Autodesk Inventor part; units mm, degrees
(part 5 of 5)
  line L3248 (77.264, 12.2136) -> (77.264, 9.6132) projected
  line L3249 (77.264, 9.6132) -> (78.0881, 9.6132) projected
  line L3250 (53.0271, 16.9127) -> (66.8267, 16.9127) projected
  line L3251 (66.8267, 16.9127) -> (66.8267, 3.113) projected
  line L3252 (53.0271, 3.113) -> (53.0271, 16.9127) projected
  line L3253 (66.8267, 3.113) -> (53.0271, 3.113) projected
  line L3254 (78.0881, 9.6132) -> (78.0881, 3.3431) projected
  line L3255 (78.7329, 22.163) -> (64.9333, 22.163) projected
  line L3256 (78.7329, 35.9625) -> (78.7329, 22.163) projected
  line L3257 (64.9333, 35.9625) -> (78.7329, 35.9625) projected
  line L3258 (69.2079, 41.2129) -> (55.4083, 41.2129) projected
  line L3259 (69.2079, 55.0125) -> (69.2079, 41.2129) projected
  line L3260 (55.4083, 55.0125) -> (69.2079, 55.0125) projected
  line L3261 (55.4083, 41.2129) -> (55.4083, 55.0125) projected
  line L3262 (50.1579, 55.0125) -> (50.1579, 41.2129) projected
  line L3263 (50.1579, 41.2129) -> (36.3583, 41.2129) projected
  line L3264 (36.3583, 55.0125) -> (50.1579, 55.0125) projected
  line L3265 (36.3583, 41.2129) -> (36.3583, 55.0125) projected
  line L3266 (84.6391, 15.4423) -> (78.0881, 15.4423) projected
  line L3267 (78.0881, 3.3431) -> (79.8132, 3.3431) projected
  line L3268 (84.6391, 3.3431) -> (84.6391, 7.8135) projected
  line L3269 (82.9137, 3.3431) -> (84.6391, 3.3431) projected
  line L3270 (82.9137, 2.1429) -> (82.9137, 3.3431) projected
  line L3271 (79.8132, 2.1429) -> (82.9137, 2.1429) projected
  line L3272 (79.8132, 3.3431) -> (79.8132, 2.1429) projected
  line L3273 (21.5828, 60.2629) -> (7.7832, 60.2629) projected
  line L3274 (7.7832, 74.0625) -> (21.5828, 74.0625) projected
  line L3275 (7.7832, 60.2629) -> (7.7832, 74.0625) projected
  line L3276 (21.5828, 74.0625) -> (21.5828, 60.2629) projected
  line L3277 (31.5957, 60.2629) -> (31.5957, 74.0625) projected
  line L3278 (35.8704, 79.3129) -> (22.0707, 79.3129) projected
  line L3279 (45.3954, 60.2629) -> (31.5957, 60.2629) projected
  line L3280 (31.5957, 74.0625) -> (45.3954, 74.0625) projected
  line L3281 (45.3954, 74.0625) -> (45.3954, 60.2629) projected
  line L3282 (0.0951, 2.187) -> (0.0951, 117.85) projected
  line L3283 (16.8203, 79.3129) -> (3.0193, 79.3129) projected
  line L3284 (3.0193, 79.3129) -> (3.0193, 93.1125) projected
  line L3285 (16.8203, 93.1125) -> (16.8203, 79.3129) projected
  line L3286 (3.0193, 93.1125) -> (16.8203, 93.1125) projected
  line L3287 (16.8203, 103.125) -> (3.0193, 103.125) projected
  line L3288 (3.0193, 103.125) -> (3.0193, 116.926) projected
  line L3289 (3.0193, 116.926) -> (16.8203, 116.926) projected
  line L3290 (16.8203, 116.926) -> (16.8203, 103.125) projected
  line L3291 (124.463, 12.2136) -> (84.6391, 12.2136) projected
  line L3292 (84.6391, 12.2136) -> (84.6391, 15.4423) projected
  line L3293 (84.6391, 7.8135) -> (124.463, 7.8135) projected
  line L3294 (97.7829, 35.9625) -> (97.7829, 22.163) projected
  line L3295 (103.033, 22.163) -> (103.033, 35.9625) projected
  line L3296 (116.833, 22.163) -> (103.033, 22.163) projected
  line L3297 (116.833, 35.9625) -> (116.833, 22.163) projected
  line L3298 (103.033, 35.9625) -> (116.833, 35.9625) projected
  line L3299 (97.7829, 22.163) -> (83.9833, 22.163) projected
  line L3300 (83.9833, 22.163) -> (83.9833, 35.9625) projected
  line L3301 (107.308, 41.2129) -> (93.5083, 41.2129) projected
  line L3302 (83.9833, 35.9625) -> (97.7829, 35.9625) projected
  line L3303 (93.5083, 55.0125) -> (107.308, 55.0125) projected
  line L3304 (93.5083, 41.2129) -> (93.5083, 55.0125) projected
  line L3305 (22.0707, 93.1125) -> (35.8704, 93.1125) projected
  line L3306 (22.0707, 79.3129) -> (22.0707, 93.1125) projected
  line L3307 (35.8704, 93.1125) -> (35.8704, 79.3129) projected
  line L3308 (41.1208, 79.3129) -> (41.1208, 93.1125) projected
  line L3309 (54.919, 79.3129) -> (41.1208, 79.3129) projected
  line L3310 (54.919, 93.1125) -> (54.919, 79.3129) projected
  line L3311 (74.4583, 41.2129) -> (74.4583, 55.0125) projected
  line L3312 (83.4954, 60.2629) -> (69.6958, 60.2629) projected
  line L3313 (69.6958, 60.2629) -> (69.6958, 74.0625) projected
  line L3314 (83.4954, 74.0625) -> (83.4954, 60.2629) projected
  line L3315 (74.4583, 55.0125) -> (88.2579, 55.0125) projected
  line L3316 (88.2579, 55.0125) -> (88.2579, 41.2129) projected
  line L3317 (88.2579, 41.2129) -> (74.4583, 41.2129) projected
  line L3318 (50.6458, 74.0625) -> (64.4454, 74.0625) projected
  line L3319 (64.4454, 74.0625) -> (64.4454, 60.2629) projected
  line L3320 (64.4454, 60.2629) -> (50.6458, 60.2629) projected
  line L3321 (50.6458, 60.2629) -> (50.6458, 74.0625) projected
  line L3322 (73.9704, 79.3129) -> (60.1694, 79.3129) projected
  line L3323 (79.2194, 79.3129) -> (79.2194, 93.1125) projected
  line L3324 (73.9704, 93.1125) -> (73.9704, 79.3129) projected
  line L3325 (60.1694, 93.1125) -> (73.9704, 93.1125) projected
  line L3326 (60.1694, 79.3129) -> (60.1694, 93.1125) projected
  line L3327 (69.6958, 74.0625) -> (83.4954, 74.0625) projected
  line L3328 (107.794, 60.2629) -> (107.794, 74.0625) projected
  line L3329 (102.545, 74.0625) -> (102.545, 60.2629) projected
  line L3330 (102.545, 60.2629) -> (88.7444, 60.2629) projected
  line L3331 (88.7444, 74.0625) -> (102.545, 74.0625) projected
  line L3332 (88.7444, 60.2629) -> (88.7444, 74.0625) projected
  line L3333 (54.919, 103.125) -> (41.1208, 103.125) projected
  line L3334 (54.919, 116.926) -> (54.919, 103.125) projected
  line L3335 (41.1208, 103.125) -> (41.1208, 116.926) projected
  line L3336 (41.1208, 116.926) -> (54.919, 116.926) projected
  line L3337 (41.1208, 93.1125) -> (54.919, 93.1125) projected
  line L3338 (0.0951, 117.85) -> (0.102, 118.007) projected
  line L3339 (0.102, 118.007) -> (0.1199, 118.163) projected
  line L3340 (0.1199, 118.163) -> (0.1502, 118.317) projected
  line L3341 (0.4768, 119.025) -> (0.5746, 119.149) projected
  line L3342 (0.39, 118.894) -> (0.4768, 119.025) projected
  line L3343 (0.3128, 118.758) -> (0.39, 118.894) projected
  line L3344 (0.248, 118.616) -> (0.3128, 118.758) projected
  line L3345 (0.1929, 118.468) -> (0.248, 118.616) projected
  line L3346 (0.1502, 118.317) -> (0.1929, 118.468) projected
  line L3347 (0.5746, 119.149) -> (0.6808, 119.265) projected
  line L3348 (0.6808, 119.265) -> (0.7965, 119.371) projected
  line L3349 (0.7965, 119.371) -> (0.9192, 119.469) projected
  line L3350 (0.9192, 119.469) -> (1.0501, 119.556) projected
  line L3351 (1.0501, 119.556) -> (1.1879, 119.633) projected
  line L3352 (1.1879, 119.633) -> (1.3298, 119.698) projected
  line L3353 (1.3298, 119.698) -> (1.4759, 119.753) projected
  line L3354 (1.4759, 119.753) -> (1.6288, 119.796) projected
  line L3355 (1.6288, 119.796) -> (1.7818, 119.826) projected
  line L3356 (1.7818, 119.826) -> (1.9389, 119.844) projected
  line L3357 (1.9389, 119.844) -> (2.096, 119.849) projected
  line L3358 (107.308, 55.0125) -> (107.308, 41.2129) projected
  line L3359 (112.558, 41.2129) -> (112.558, 55.0125) projected
  line L3360 (126.358, 41.2129) -> (112.558, 41.2129) projected
  line L3361 (126.358, 55.0125) -> (126.358, 41.2129) projected
  line L3362 (112.558, 55.0125) -> (126.358, 55.0125) projected
  line L3363 (121.595, 60.2629) -> (107.794, 60.2629) projected
  line L3364 (107.794, 74.0625) -> (121.595, 74.0625) projected
  line L3365 (121.595, 74.0625) -> (121.595, 60.2629) projected
  line L3366 (93.0204, 79.3129) -> (79.2194, 79.3129) projected
  line L3367 (93.0204, 93.1125) -> (93.0204, 79.3129) projected
  line L3368 (79.2194, 93.1125) -> (93.0204, 93.1125) projected
  line L3369 (93.0204, 103.125) -> (79.2194, 103.125) projected
  line L3370 (98.2694, 103.125) -> (98.2694, 116.926) projected
  line L3371 (145.896, 74.0625) -> (159.695, 74.0625) projected
  line L3372 (159.695, 74.0625) -> (159.695, 60.2629) projected
  line L3373 (145.896, 60.2629) -> (145.896, 74.0625) projected
  line L3374 (140.645, 74.0625) -> (140.645, 60.2629) projected
  line L3375 (140.645, 60.2629) -> (126.846, 60.2629) projected
  line L3376 (126.846, 74.0625) -> (140.645, 74.0625) projected
  line L3377 (126.846, 60.2629) -> (126.846, 74.0625) projected
  line L3378 (112.07, 79.3129) -> (98.2694, 79.3129) projected
  line L3379 (98.2694, 93.1125) -> (112.07, 93.1125) projected
  line L3380 (98.2694, 79.3129) -> (98.2694, 93.1125) projected
  line L3381 (131.12, 79.3129) -> (117.321, 79.3129) projected
  line L3382 (112.07, 93.1125) -> (112.07, 79.3129) projected
  line L3383 (117.321, 79.3129) -> (117.321, 93.1125) projected
  line L3384 (131.12, 93.1125) -> (131.12, 79.3129) projected
  line L3385 (117.321, 93.1125) -> (131.12, 93.1125) projected
  line L3386 (79.2194, 116.926) -> (93.0204, 116.926) projected
  line L3387 (93.0204, 116.926) -> (93.0204, 103.125) projected
  line L3388 (79.2194, 103.125) -> (79.2194, 116.926) projected
  line L3389 (73.9704, 103.125) -> (60.1694, 103.125) projected
  line L3390 (73.9704, 116.926) -> (73.9704, 103.125) projected
  line L3391 (60.1694, 103.125) -> (60.1694, 116.926) projected
  line L3392 (60.1694, 116.926) -> (73.9704, 116.926) projected
  line L3393 (141.133, 22.163) -> (141.133, 35.9625) projected
  line L3394 (141.133, 35.9625) -> (154.933, 35.9625) projected
  line L3395 (138.264, 7.8135) -> (178.088, 7.8135) projected
  line L3396 (178.088, 12.2136) -> (138.264, 12.2136) projected
  line L3397 (154.933, 35.9625) -> (154.933, 22.163) projected
  line L3398 (178.088, 15.4423) -> (178.088, 12.2136) projected
  line L3399 (160.183, 22.163) -> (160.183, 35.9625) projected
  line L3400 (173.983, 22.163) -> (160.183, 22.163) projected
  line L3401 (160.183, 35.9625) -> (173.983, 35.9625) projected
  line L3402 (173.983, 35.9625) -> (173.983, 22.163) projected
  line L3403 (184.638, 12.2136) -> (184.638, 15.4423) projected
  line L3404 (184.638, 15.4423) -> (178.088, 15.4423) projected
  line L3405 (193.033, 22.163) -> (179.233, 22.163) projected
  line L3406 (179.233, 22.163) -> (179.233, 35.9625) projected
  line L3407 (179.233, 35.9625) -> (193.033, 35.9625) projected
  line L3408 (193.033, 35.9625) -> (193.033, 22.163) projected
  line L3409 (178.088, 7.8135) -> (178.088, 3.3431) projected
  line L3410 (178.088, 3.3431) -> (179.813, 3.3431) projected
  line L3411 (179.813, 3.3431) -> (179.813, 2.1429) projected
  line L3412 (179.813, 2.1429) -> (182.914, 2.1429) projected
  line L3413 (182.914, 2.1429) -> (182.914, 3.3431) projected
  line L3414 (185.463, 12.2136) -> (184.638, 12.2136) projected
  line L3415 (185.463, 9.6132) -> (185.463, 12.2136) projected
  line L3416 (184.638, 9.6132) -> (185.463, 9.6132) projected
  line L3417 (184.638, 3.3431) -> (184.638, 9.6132) projected
  line L3418 (182.914, 3.3431) -> (184.638, 3.3431) projected
  line L3419 (195.902, 16.9127) -> (209.702, 16.9127) projected
  line L3420 (209.702, 16.9127) -> (209.702, 3.113) projected
  line L3421 (209.702, 3.113) -> (195.902, 3.113) projected
  line L3422 (195.902, 3.113) -> (195.902, 16.9127) projected
  line L3423 (124.463, 16.9127) -> (124.463, 12.2136) projected
  line L3424 (124.463, 7.8135) -> (124.463, 3.113) projected
  line L3425 (124.463, 3.113) -> (138.264, 3.113) projected
  line L3426 (138.264, 12.2136) -> (138.264, 16.9127) projected
  line L3427 (138.264, 16.9127) -> (124.463, 16.9127) projected
  line L3428 (122.083, 35.9625) -> (135.883, 35.9625) projected
  line L3429 (135.883, 22.163) -> (122.083, 22.163) projected
  line L3430 (122.083, 22.163) -> (122.083, 35.9625) projected
  line L3431 (135.883, 35.9625) -> (135.883, 22.163) projected
  line L3432 (138.264, 3.113) -> (138.264, 7.8135) projected
  line L3433 (154.933, 22.163) -> (141.133, 22.163) projected
  line L3434 (202.558, 41.2129) -> (188.758, 41.2129) projected
  line L3435 (188.758, 41.2129) -> (188.758, 55.0125) projected
  line L3436 (188.758, 55.0125) -> (202.558, 55.0125) projected
  line L3437 (202.558, 55.0125) -> (202.558, 41.2129) projected
  line L3438 (221.608, 55.0125) -> (221.608, 41.2129) projected
  line L3439 (226.858, 41.2129) -> (226.858, 55.0125) projected
  line L3440 (240.658, 41.2129) -> (226.858, 41.2129) projected
  line L3441 (240.658, 55.0125) -> (240.658, 41.2129) projected
  line L3442 (257.813, 55.0125) -> (257.813, 50.3135) projected
  line L3443 (257.813, 50.3135) -> (256.089, 50.3135) projected
  line L3444 (256.089, 50.3135) -> (256.089, 53.5421) projected
  line L3445 (256.089, 53.5421) -> (249.538, 53.5421) projected
  line L3446 (248.714, 47.7132) -> (249.538, 47.7132) projected
  line L3447 (249.538, 50.3135) -> (248.714, 50.3135) projected
  line L3448 (248.714, 50.3135) -> (248.714, 47.7132) projected
  line L3449 (249.538, 53.5421) -> (249.538, 50.3135) projected
  line L3450 (257.813, 45.9133) -> (257.813, 41.2129) projected
  line L3451 (256.089, 45.9133) -> (257.813, 45.9133) projected
  line L3452 (257.813, 41.2129) -> (271.614, 41.2129) projected
  line L3453 (256.089, 41.4433) -> (256.089, 45.9133) projected
  line L3454 (271.614, 45.9133) -> (273.338, 45.9133) projected
  line L3455 (273.338, 45.9133) -> (273.338, 41.4433) projected
  line L3456 (273.338, 41.4433) -> (275.063, 41.4433) projected
  line L3457 (271.614, 41.2129) -> (271.614, 45.9133) projected
  line L3458 (273.338, 50.3135) -> (271.614, 50.3135) projected
  line L3459 (271.614, 50.3135) -> (271.614, 55.0125) projected
  line L3460 (273.338, 53.5421) -> (273.338, 50.3135) projected
  line L3461 (278.758, 60.2629) -> (264.958, 60.2629) projected
  line L3462 (271.614, 55.0125) -> (257.813, 55.0125) projected
  line L3463 (278.758, 74.0625) -> (278.758, 60.2629) projected
  line L3464 (264.958, 74.0625) -> (278.758, 74.0625) projected
  line L3465 (264.958, 60.2629) -> (264.958, 74.0625) projected
  line L3466 (260.196, 79.3129) -> (273.995, 79.3129) projected
  line L3467 (150.17, 79.3129) -> (136.371, 79.3129) projected
  line L3468 (169.22, 79.3129) -> (155.421, 79.3129) projected
  line L3469 (136.371, 93.1125) -> (150.17, 93.1125) projected
  line L3470 (136.371, 79.3129) -> (136.371, 93.1125) projected
  line L3471 (150.17, 93.1125) -> (150.17, 79.3129) projected
  line L3472 (155.421, 79.3129) -> (155.421, 93.1125) projected
  line L3473 (169.22, 93.1125) -> (169.22, 79.3129) projected
  line L3474 (155.421, 93.1125) -> (169.22, 93.1125) projected
  line L3475 (173.983, 103.125) -> (160.183, 103.125) projected
  line L3476 (154.933, 103.125) -> (141.133, 103.125) projected
  line L3477 (141.133, 103.125) -> (141.133, 116.926) projected
  line L3478 (141.133, 116.926) -> (154.933, 116.926) projected
  line L3479 (154.933, 116.926) -> (154.933, 103.125) projected
  line L3480 (160.183, 103.125) -> (160.183, 116.926) projected
  line L3481 (160.183, 116.926) -> (173.983, 116.926) projected
  line L3482 (173.983, 116.926) -> (173.983, 103.125) projected
  line L3483 (178.745, 74.0625) -> (178.745, 60.2629) projected
  line L3484 (178.745, 60.2629) -> (164.946, 60.2629) projected
  line L3485 (164.946, 60.2629) -> (164.946, 74.0625) projected
  line L3486 (164.946, 74.0625) -> (178.745, 74.0625) projected
  line L3487 (197.795, 60.2629) -> (183.996, 60.2629) projected
  line L3488 (197.795, 74.0625) -> (197.795, 60.2629) projected
  line L3489 (183.996, 60.2629) -> (183.996, 74.0625) projected
  line L3490 (183.996, 74.0625) -> (197.795, 74.0625) projected
  line L3491 (183.508, 55.0125) -> (183.508, 41.2129) projected
  line L3492 (183.508, 41.2129) -> (169.708, 41.2129) projected
  line L3493 (169.708, 41.2129) -> (169.708, 55.0125) projected
  line L3494 (169.708, 55.0125) -> (183.508, 55.0125) projected
  line L3495 (188.27, 79.3129) -> (174.471, 79.3129) projected
  line L3496 (207.32, 79.3129) -> (193.521, 79.3129) projected
  line L3497 (174.471, 93.1125) -> (188.27, 93.1125) projected
  line L3498 (174.471, 79.3129) -> (174.471, 93.1125) projected
  line L3499 (188.27, 93.1125) -> (188.27, 79.3129) projected
  line L3500 (193.521, 79.3129) -> (193.521, 93.1125) projected
  line L3501 (207.32, 93.1125) -> (207.32, 79.3129) projected
  line L3502 (193.521, 93.1125) -> (207.32, 93.1125) projected
  line L3503 (216.845, 74.0625) -> (216.845, 60.2629) projected
  line L3504 (216.845, 60.2629) -> (203.046, 60.2629) projected
  line L3505 (203.046, 60.2629) -> (203.046, 74.0625) projected
  line L3506 (203.046, 74.0625) -> (216.845, 74.0625) projected
  line L3507 (216.845, 103.125) -> (203.046, 103.125) projected
  line L3508 (193.033, 103.125) -> (179.233, 103.125) projected
  line L3509 (179.233, 103.125) -> (179.233, 116.926) projected
  line L3510 (179.233, 116.926) -> (193.033, 116.926) projected
  line L3511 (193.033, 116.926) -> (193.033, 103.125) projected
  line L3512 (203.046, 103.125) -> (203.046, 116.926) projected
  line L3513 (216.845, 116.926) -> (216.845, 103.125) projected
  line L3514 (203.046, 116.926) -> (216.845, 116.926) projected
  line L3515 (235.895, 60.2629) -> (222.096, 60.2629) projected
  line L3516 (222.096, 60.2629) -> (222.096, 74.0625) projected
  line L3517 (222.096, 74.0625) -> (235.895, 74.0625) projected
  line L3518 (235.895, 74.0625) -> (235.895, 60.2629) projected
  line L3519 (226.858, 55.0125) -> (240.658, 55.0125) projected
  line L3520 (198.283, 35.9625) -> (212.083, 35.9625) projected
  line L3521 (212.083, 35.9625) -> (212.083, 22.163) projected
  line L3522 (212.083, 22.163) -> (198.283, 22.163) projected
  line L3523 (207.808, 55.0125) -> (221.608, 55.0125) projected
  line L3524 (207.808, 41.2129) -> (207.808, 55.0125) projected
  line L3525 (217.333, 35.9625) -> (231.133, 35.9625) projected
  line L3526 (231.133, 35.9625) -> (231.133, 22.163) projected
  line L3527 (231.133, 22.163) -> (217.333, 22.163) projected
  line L3528 (221.608, 41.2129) -> (207.808, 41.2129) projected
  line L3529 (198.283, 22.163) -> (198.283, 35.9625) projected
  line L3530 (217.333, 22.163) -> (217.333, 35.9625) projected
  line L3531 (226.37, 79.3129) -> (212.571, 79.3129) projected
  line L3532 (245.42, 79.3129) -> (231.621, 79.3129) projected
  line L3533 (212.571, 93.1125) -> (226.37, 93.1125) projected
  line L3534 (212.571, 79.3129) -> (212.571, 93.1125) projected
  line L3535 (226.37, 93.1125) -> (226.37, 79.3129) projected
  line L3536 (231.621, 79.3129) -> (231.621, 93.1125) projected
  line L3537 (245.42, 93.1125) -> (245.42, 79.3129) projected
  line L3538 (231.621, 93.1125) -> (245.42, 93.1125) projected
  line L3539 (235.895, 103.125) -> (222.096, 103.125) projected
  line L3540 (254.945, 103.125) -> (241.146, 103.125) projected
  line L3541 (241.146, 116.926) -> (254.945, 116.926) projected
  line L3542 (241.146, 103.125) -> (241.146, 116.926) projected
  line L3543 (222.096, 103.125) -> (222.096, 116.926) projected
  line L3544 (222.096, 116.926) -> (235.895, 116.926) projected
  line L3545 (235.895, 116.926) -> (235.895, 103.125) projected
  line L3546 (241.146, 74.0625) -> (254.945, 74.0625) projected
  line L3547 (254.945, 74.0625) -> (254.945, 60.2629) projected
  line L3548 (254.945, 60.2629) -> (241.146, 60.2629) projected
  line L3549 (241.146, 60.2629) -> (241.146, 74.0625) projected
  line L3550 (251.92, 85.8132) -> (251.92, 79.5433) projected
  line L3551 (251.92, 79.5433) -> (253.646, 79.5433) projected
  line L3552 (256.745, 78.3428) -> (256.745, 79.5433) projected
  line L3553 (253.646, 79.5433) -> (253.646, 78.3428) projected
  line L3554 (253.646, 78.3428) -> (256.745, 78.3428) projected
  line L3555 (256.745, 79.5433) -> (258.47, 79.5433) projected
  line L3556 (260.196, 84.0133) -> (260.196, 79.3129) projected
  line L3557 (258.47, 84.0133) -> (260.196, 84.0133) projected
  line L3558 (258.47, 79.5433) -> (258.47, 84.0133) projected
  line L3559 (260.196, 93.1125) -> (260.196, 88.4135) projected
  line L3560 (260.196, 88.4135) -> (258.47, 88.4135) projected
  line L3561 (251.095, 85.8132) -> (251.92, 85.8132) projected
  line L3562 (251.095, 88.4135) -> (251.095, 85.8132) projected
  line L3563 (251.92, 88.4135) -> (251.095, 88.4135) projected
  line L3564 (251.92, 91.6421) -> (251.92, 88.4135) projected
  line L3565 (258.47, 91.6421) -> (251.92, 91.6421) projected
  line L3566 (258.47, 88.4135) -> (258.47, 91.6421) projected
  line L3567 (273.995, 93.1125) -> (260.196, 93.1125) projected
  line L3568 (273.995, 103.125) -> (260.196, 103.125) projected
  line L3569 (273.995, 116.926) -> (273.995, 103.125) projected
  line L3570 (260.196, 116.926) -> (273.995, 116.926) projected
  line L3571 (260.196, 103.125) -> (260.196, 116.926) projected
  line L3572 (254.945, 116.926) -> (254.945, 103.125) projected
  line L3573 (249.538, 47.7132) -> (249.538, 41.4433) projected
  line L3574 (249.538, 41.4433) -> (251.263, 41.4433) projected
  line L3575 (251.263, 41.4433) -> (251.263, 40.2428) projected
  line L3576 (251.263, 40.2428) -> (254.362, 40.2428) projected
  line L3577 (254.362, 40.2428) -> (254.362, 41.4433) projected
  line L3578 (254.362, 41.4433) -> (256.089, 41.4433) projected
  line L3579 (164.458, 41.2129) -> (150.658, 41.2129) projected
  line L3580 (164.458, 55.0125) -> (164.458, 41.2129) projected
  line L3581 (150.658, 55.0125) -> (164.458, 55.0125) projected
  line L3582 (150.658, 41.2129) -> (150.658, 55.0125) projected
  line L3583 (159.695, 60.2629) -> (145.896, 60.2629) projected
  line L3584 (145.408, 55.0125) -> (145.408, 41.2129) projected
  line L3585 (145.408, 41.2129) -> (131.608, 41.2129) projected
  line L3586 (131.608, 55.0125) -> (145.408, 55.0125) projected
  line L3587 (131.608, 41.2129) -> (131.608, 55.0125) projected
  line L3588 (0.7965, 0.6656) -> (0.6808, 0.7731) projected
  line L3589 (0.6808, 0.7731) -> (0.5746, 0.8875) projected
  line L3590 (0.5746, 0.8875) -> (0.4768, 1.0115) projected
  line L3591 (0.4768, 1.0115) -> (0.39, 1.1424) projected
  line L3592 (0.39, 1.1424) -> (0.3128, 1.2788) projected
  line L3593 (0.3128, 1.2788) -> (0.248, 1.4221) projected
  line L3594 (14.9269, 35.9625) -> (14.9269, 31.2636) projected
  line L3595 (14.9269, 31.2636) -> (13.2016, 31.2636) projected
  line L3596 (13.2016, 31.2636) -> (13.2016, 34.4923) projected
  line L3597 (13.2016, 34.4923) -> (6.6518, 34.4923) projected
  line L3598 (6.6518, 34.4923) -> (6.6518, 31.2636) projected
  line L3599 (6.6518, 31.2636) -> (5.8263, 31.2636) projected
  line L3600 (5.8263, 31.2636) -> (5.8263, 28.6632) projected
  line L3601 (5.8263, 28.6632) -> (6.6518, 28.6632) projected
  line L3602 (30.4519, 26.8635) -> (30.4519, 22.3931) projected
  line L3603 (30.4519, 22.3931) -> (32.1758, 22.3931) projected
  line L3604 (32.1758, 22.3931) -> (32.1758, 21.1928) projected
  line L3605 (32.1758, 21.1928) -> (35.2764, 21.1928) projected
  line L3606 (35.2764, 21.1928) -> (35.2764, 22.3931) projected
  line L3607 (35.2764, 22.3931) -> (37.0018, 22.3931) projected
  line L3608 (37.0018, 22.3931) -> (37.0018, 28.6632) projected
  line L3609 (37.0018, 28.6632) -> (37.8273, 28.6632) projected
  line L3610 (37.8273, 28.6632) -> (37.8273, 31.2636) projected
  line L3611 (37.8273, 31.2636) -> (37.0018, 31.2636) projected
  line L3612 (37.0018, 31.2636) -> (37.0018, 34.4923) projected
  line L3613 (37.0018, 34.4923) -> (30.4519, 34.4923) projected
  line L3614 (30.4519, 31.2636) -> (28.7266, 31.2636) projected
  line L3615 (28.7266, 31.2636) -> (28.7266, 35.9625) projected
  line L3616 (30.4519, 34.4923) -> (30.4519, 31.2636) projected
  line L3617 (13.2016, 26.8635) -> (14.9269, 26.8635) projected
  line L3618 (13.2016, 22.3931) -> (13.2016, 26.8635) projected
  line L3619 (6.6518, 28.6632) -> (6.6518, 22.3931) projected
  line L3620 (6.6518, 22.3931) -> (8.3771, 22.3931) projected
  line L3621 (29.213, 16.9127) -> (43.0142, 16.9127) projected
  line L3622 (43.0142, 16.9127) -> (43.0142, 3.113) projected
  line L3623 (43.0142, 3.113) -> (29.213, 3.113) projected
  line L3624 (29.213, 3.113) -> (29.213, 16.9127) projected
  line L3625 (14.9269, 26.8635) -> (14.9269, 22.163) projected
  line L3626 (14.9269, 22.163) -> (28.7266, 22.163) projected
  line L3627 (28.7266, 22.163) -> (28.7266, 26.8635) projected
  line L3628 (28.7266, 26.8635) -> (30.4519, 26.8635) projected
  line L3629 (8.3771, 22.3931) -> (8.3771, 21.1928) projected
  line L3630 (11.4763, 21.1928) -> (11.4763, 22.3931) projected
  line L3631 (8.3771, 21.1928) -> (11.4763, 21.1928) projected
  line L3632 (5.4019, 16.9127) -> (19.2016, 16.9127) projected
  line L3633 (5.4019, 3.113) -> (5.4019, 16.9127) projected
  line L3634 (19.2016, 3.113) -> (5.4019, 3.113) projected
  line L3635 (19.2016, 16.9127) -> (19.2016, 3.113) projected
  line L3636 (11.4763, 22.3931) -> (13.2016, 22.3931) projected
  line L3637 (0.248, 1.4221) -> (0.1929, 1.5696) projected
  line L3638 (0.1929, 1.5696) -> (0.1502, 1.7198) projected
  line L3639 (0.1502, 1.7198) -> (0.1199, 1.8741) projected
  line L3640 (0.1199, 1.8741) -> (0.102, 2.0298) projected
  line L3641 (0.102, 2.0298) -> (0.0951, 2.187) projected
  line L3642 (2.096, 0.1874) -> (1.9389, 0.1929) projected
  line L3643 (1.9389, 0.1929) -> (1.7818, 0.2122) projected
  line L3644 (1.7818, 0.2122) -> (1.6288, 0.2425) projected
  line L3645 (0.9192, 0.5691) -> (0.7965, 0.6656) projected
  line L3646 (1.0501, 0.4823) -> (0.9192, 0.5691) projected
  line L3647 (1.3298, 0.339) -> (1.1879, 0.4051) projected
  line L3648 (1.4759, 0.2853) -> (1.3298, 0.339) projected
  line L3649 (1.6288, 0.2425) -> (1.4759, 0.2853) projected
  line L3650 (1.1879, 0.4051) -> (1.0501, 0.4823) projected
  line L3651 (64.9333, 22.163) -> (64.9333, 35.9625) projected
  line L3652 (59.6829, 35.9625) -> (59.6829, 22.163) projected
  line L3653 (59.6829, 22.163) -> (45.8833, 22.163) projected
  line L3654 (45.8833, 22.163) -> (45.8833, 35.9625) projected
  line L3655 (45.8833, 35.9625) -> (59.6829, 35.9625) projected
  line L3656 (288.771, 35.9625) -> (302.57, 35.9625) projected
  line L3657 (302.57, 35.9625) -> (302.57, 22.163) projected
  line L3658 (288.771, 22.163) -> (288.771, 35.9625) projected
  line L3659 (283.52, 22.163) -> (269.721, 22.163) projected
  line L3660 (269.721, 35.9625) -> (283.52, 35.9625) projected
  line L3661 (269.721, 22.163) -> (269.721, 35.9625) projected
  line L3662 (283.52, 35.9625) -> (283.52, 22.163) projected
  line L3663 (269.721, 16.9127) -> (283.52, 16.9127) projected
  line L3664 (283.52, 16.9127) -> (283.52, 3.113) projected
  line L3665 (283.52, 3.113) -> (269.721, 3.113) projected
  line L3666 (269.721, 3.113) -> (269.721, 16.9127) projected
  line L3667 (302.57, 22.163) -> (288.771, 22.163) projected
  line L3668 (288.771, 16.9127) -> (302.57, 16.9127) projected
  line L3669 (288.771, 3.113) -> (288.771, 16.9127) projected
  line L3670 (302.57, 16.9127) -> (302.57, 3.113) projected
  line L3671 (302.57, 3.113) -> (288.771, 3.113) projected
  line L3672 (302.57, 41.2129) -> (288.771, 41.2129) projected
  line L3673 (279.888, 47.7132) -> (280.713, 47.7132) projected
  line L3674 (280.713, 50.3135) -> (279.888, 50.3135) projected
  line L3675 (280.713, 47.7132) -> (280.713, 50.3135) projected
  line L3676 (279.888, 50.3135) -> (279.888, 53.5421) projected
  line L3677 (288.771, 41.2129) -> (288.771, 55.0125) projected
  line L3678 (302.57, 55.0125) -> (302.57, 41.2129) projected
  line L3679 (219.713, 16.9127) -> (233.514, 16.9127) projected
  line L3680 (233.514, 16.9127) -> (233.514, 3.113) projected
  line L3681 (233.514, 3.113) -> (219.713, 3.113) projected
  line L3682 (219.713, 3.113) -> (219.713, 16.9127) projected
  line L3683 (250.671, 16.9127) -> (264.47, 16.9127) projected
  line L3684 (264.47, 16.9127) -> (264.47, 3.113) projected
  line L3685 (264.47, 3.113) -> (250.671, 3.113) projected
  line L3686 (250.671, 3.113) -> (250.671, 16.9127) projected
  line L3687 (288.771, 55.0125) -> (302.57, 55.0125) projected
  line L3688 (302.57, 60.2629) -> (288.771, 60.2629) projected
  line L3689 (288.771, 60.2629) -> (288.771, 74.0625) projected
  line L3690 (302.57, 74.0625) -> (302.57, 60.2629) projected
  line L3691 (288.771, 74.0625) -> (302.57, 74.0625) projected
  line L3692 (277.446, 78.3428) -> (280.545, 78.3428) projected
  line L3693 (277.446, 79.5433) -> (277.446, 78.3428) projected
  line L3694 (275.721, 79.5433) -> (277.446, 79.5433) projected
  line L3695 (273.995, 79.3129) -> (273.995, 84.0133) projected
  line L3696 (273.995, 84.0133) -> (275.721, 84.0133) projected
  line L3697 (275.721, 84.0133) -> (275.721, 79.5433) projected
  line L3698 (282.271, 88.4135) -> (282.271, 91.6421) projected
  line L3699 (275.721, 88.4135) -> (273.995, 88.4135) projected
  line L3700 (275.721, 91.6421) -> (275.721, 88.4135) projected
  line L3701 (273.995, 88.4135) -> (273.995, 93.1125) projected
  line L3702 (282.271, 91.6421) -> (275.721, 91.6421) projected
  line L3703 (280.545, 79.5433) -> (282.271, 79.5433) projected
  line L3704 (282.271, 79.5433) -> (282.271, 85.8132) projected
  line L3705 (282.271, 85.8132) -> (283.096, 85.8132) projected
  line L3706 (283.096, 88.4135) -> (282.271, 88.4135) projected
  line L3707 (283.096, 85.8132) -> (283.096, 88.4135) projected
  line L3708 (280.545, 78.3428) -> (280.545, 79.5433) projected
  line L3709 (243.527, 35.9625) -> (257.327, 35.9625) projected
  line L3710 (257.327, 35.9625) -> (257.327, 22.163) projected
  line L3711 (257.327, 22.163) -> (243.527, 22.163) projected
  line L3712 (243.527, 22.163) -> (243.527, 35.9625) projected
  line L3713 (279.888, 41.4433) -> (279.888, 47.7132) projected
  line L3714 (278.164, 41.4433) -> (279.888, 41.4433) projected
  line L3715 (279.888, 53.5421) -> (273.338, 53.5421) projected
  line L3716 (275.063, 41.4433) -> (275.063, 40.2428) projected
  line L3717 (275.063, 40.2428) -> (278.164, 40.2428) projected
  line L3718 (278.164, 40.2428) -> (278.164, 41.4433) projected
  line L3719 (303.496, 119.849) -> (303.652, 119.844) projected
  line L3720 (288.771, 79.3129) -> (288.771, 93.1125) projected
  line L3721 (288.771, 93.1125) -> (302.57, 93.1125) projected
  line L3722 (302.57, 93.1125) -> (302.57, 79.3129) projected
  line L3723 (302.57, 79.3129) -> (288.771, 79.3129) projected
  line L3724 (3.0193, 116.926) -> (16.8203, 116.926)
  line L3725 (16.8203, 116.926) -> (16.8203, 103.125)
  line L3726 (16.8203, 103.125) -> (3.0193, 103.125)
  line L3727 (3.0193, 103.125) -> (3.0193, 116.926)
  line L3728 (0.3948, 100.5005) -> (19.4448, 100.5005)
  line L3729 (19.4448, 100.5005) -> (19.4448, 119.5505)
  line L3730 (19.4448, 119.5505) -> (0.3948, 119.5505)
  line L3731 (0.3948, 119.5505) -> (0.3948, 100.5005)
  line L3732 (0.3948, 100.5005) -> (19.4448, 119.5505) construction
  line L3733 (19.4448, 100.5005) -> (0.3948, 119.5505) construction
  line L3734 (16.8203, 93.1125) -> (3.0193, 93.1125)
  line L3735 (3.0193, 93.1125) -> (3.0193, 79.3129)
  line L3736 (3.0193, 79.3129) -> (16.8203, 79.3129)
  line L3737 (16.8203, 79.3129) -> (16.8203, 93.1125)
  line L3738 (0.3948, 76.6877) -> (19.4448, 76.6877)
  line L3739 (19.4448, 76.6877) -> (19.4448, 95.7377)
  line L3740 (19.4448, 95.7377) -> (0.3948, 95.7377)
  line L3741 (0.3948, 95.7377) -> (0.3948, 76.6877)
  line L3742 (0.3948, 76.6877) -> (19.4448, 95.7377) construction
  line L3743 (19.4448, 76.6877) -> (0.3948, 95.7377) construction
  line L3744 (19.4448, 95.7377) -> (248.0448, 95.7377)
  line L3745 (248.0448, 95.7377) -> (248.0448, 76.6877)
  line L3746 (248.0448, 76.6877) -> (19.4448, 76.6877)
  line L3747 (19.4448, 76.6877) -> (19.4448, 95.7377)
  line L3748 (288.771, 93.1125) -> (302.57, 93.1125)
  line L3749 (302.57, 93.1125) -> (302.57, 79.3129)
  line L3750 (302.57, 79.3129) -> (288.771, 79.3129)
  line L3751 (288.771, 79.3129) -> (288.771, 93.1125)
  line L3752 (286.1455, 76.6877) -> (305.1955, 76.6877)
  line L3753 (305.1955, 76.6877) -> (305.1955, 95.7377)
  line L3754 (305.1955, 95.7377) -> (286.1455, 95.7377)
  line L3755 (286.1455, 95.7377) -> (286.1455, 76.6877)
  line L3756 (286.1455, 76.6877) -> (305.1955, 95.7377) construction
  line L3757 (305.1955, 76.6877) -> (286.1455, 95.7377) construction
  line L3758 (286.1455, 95.7377) -> (248.0448, 95.7377)
  line L3759 (248.0448, 95.7377) -> (248.0448, 76.6877)
  line L3760 (248.0448, 76.6877) -> (286.1455, 76.6877)
  line L3761 (286.1455, 76.6877) -> (286.1455, 95.7377)
  line L3762 (0.3948, 76.6877) -> (305.1948, 76.6877)
  line L3763 (305.1948, 76.6877) -> (305.1948, 0.4877)
  line L3764 (305.1948, 0.4877) -> (0.3948, 0.4877)
  line L3765 (0.3948, 0.4877) -> (0.3948, 76.6877)
  line L3766 (41.1208, 116.926) -> (54.919, 116.926)
  line L3767 (54.919, 116.926) -> (54.919, 103.125)
  line L3768 (54.919, 103.125) -> (41.1208, 103.125)
  line L3769 (41.1208, 103.125) -> (41.1208, 116.926)
  line L3770 (57.5449, 100.5005) -> (38.4949, 100.5005)
  line L3771 (38.4949, 100.5005) -> (38.4949, 119.5505)
  line L3772 (38.4949, 119.5505) -> (57.5449, 119.5505)
  line L3773 (57.5449, 119.5505) -> (57.5449, 100.5005)
  line L3774 (57.5449, 100.5005) -> (38.4949, 119.5505) construction
  line L3775 (38.4949, 100.5005) -> (57.5449, 119.5505) construction
  line L3776 (57.5449, 119.5505) -> (114.6949, 119.5505)
  line L3777 (114.6949, 119.5505) -> (114.6949, 100.5005)
  line L3778 (114.6949, 100.5005) -> (57.5449, 100.5005)
  line L3779 (57.5449, 100.5005) -> (57.5449, 119.5505)
  line L3780 (119.458, 100.5005) -> (138.508, 100.5005)
  line L3781 (138.508, 100.5005) -> (138.508, 119.5505)
  line L3782 (138.508, 119.5505) -> (119.458, 119.5505)
  line L3783 (119.458, 119.5505) -> (119.458, 100.5005)
  line L3784 (119.458, 100.5005) -> (138.508, 119.5505) construction
  line L3785 (138.508, 100.5005) -> (119.458, 119.5505) construction
  line L3786 (138.508, 119.5505) -> (195.658, 119.5505)
  line L3787 (195.658, 119.5505) -> (195.658, 100.5005)
  line L3788 (195.658, 100.5005) -> (138.508, 100.5005)
  line L3789 (138.508, 100.5005) -> (138.508, 119.5505)
  line L3790 (200.4205, 100.5005) -> (219.4705, 100.5005)
  line L3791 (219.4705, 100.5005) -> (219.4705, 119.5505)
  line L3792 (219.4705, 119.5505) -> (200.4205, 119.5505)
  line L3793 (200.4205, 119.5505) -> (200.4205, 100.5005)
  line L3794 (200.4205, 100.5005) -> (219.4705, 119.5505) construction
  line L3795 (219.4705, 100.5005) -> (200.4205, 119.5505) construction
  line L3796 (219.4705, 119.5505) -> (276.6205, 119.5505)
  line L3797 (276.6205, 119.5505) -> (276.6205, 100.5005)
  line L3798 (276.6205, 100.5005) -> (219.4705, 100.5005)
  line L3799 (219.4705, 100.5005) -> (219.4705, 119.5505)
  line L3800 (214.7085, 0.4878) -> (238.5185, 0.4878)
  line L3801 (238.5185, 0.4878) -> (238.5185, 19.5378)
  line L3802 (238.5185, 19.5378) -> (214.7085, 19.5378)
  line L3803 (214.7085, 19.5378) -> (214.7085, 0.4878)
  line L3804 (214.7085, 0.4878) -> (238.5185, 19.5378) construction
  line L3805 (238.5185, 0.4878) -> (214.7085, 19.5378) construction
  line L3806 (195.902, 16.9127) -> (209.702, 16.9127)
  line L3807 (209.702, 16.9127) -> (209.702, 3.113)
  line L3808 (209.702, 3.113) -> (195.902, 3.113)
  line L3809 (195.902, 3.113) -> (195.902, 16.9127)
  line L3810 (190.897, 0.4878) -> (214.707, 0.4878)
  line L3811 (214.707, 0.4878) -> (214.707, 19.5378)
  line L3812 (214.707, 19.5378) -> (190.897, 19.5378)
  line L3813 (190.897, 19.5378) -> (190.897, 0.4878)
  line L3814 (190.897, 0.4878) -> (214.707, 19.5378) construction
  line L3815 (214.707, 0.4878) -> (190.897, 19.5378) construction
  line L3816 (264.47, 16.9127) -> (250.671, 16.9127)
  line L3817 (250.671, 16.9127) -> (250.671, 3.113)
  line L3818 (250.671, 3.113) -> (264.47, 3.113)
  line L3819 (264.47, 3.113) -> (264.47, 16.9127)
  line L3820 (248.0455, 0.4878) -> (267.0955, 0.4878)
  line L3821 (267.0955, 0.4878) -> (267.0955, 19.5378)
  line L3822 (267.0955, 19.5378) -> (248.0455, 19.5378)
  line L3823 (248.0455, 19.5378) -> (248.0455, 0.4878)
  line L3824 (248.0455, 0.4878) -> (267.0955, 19.5378) construction
  line L3825 (267.0955, 0.4878) -> (248.0455, 19.5378) construction
  line L3826 (248.0455, 19.5378) -> (238.5185, 19.5378)
  line L3827 (238.5185, 19.5378) -> (238.5185, 0.4878)
  line L3828 (238.5185, 0.4878) -> (248.0455, 0.4878)
  line L3829 (248.0455, 0.4878) -> (248.0455, 19.5378)
  point P0 (0, 0)
  point P1 (0, 0)
  point P2 (9.9198, 110.0255)
  point P3 (9.9198, 86.2127)
  point P4 (295.6705, 86.2127)
  point P5 (48.0199, 110.0255)
  point P6 (128.983, 110.0255)
  point P7 (209.9455, 110.0255)
  point P8 (226.6135, 10.0128)
  point P9 (202.802, 10.0128)
  point P10 (257.5705, 10.0128)
  point P11 (0.3948, 118.9013)
  point P12 (0.3948, 1.1351)
  point P13 (305.1948, 1.133)
  point P14 (1.0418, 119.5505)
  dimension "d2" = 19.05
  dimension "d3" = 19.05
  dimension "d4" = 19.05
  dimension "d5" = 19.05
  dimension "d6" = 228.6
  dimension "d7" = 19.05
  dimension "d8" = 19.05
  dimension "d9" = 19.05
  dimension "d10" = 304.8
  dimension "d11" = 76.2
  dimension "d12" = 19.05
  dimension "d13" = 19.05
  dimension "d14" = 57.15
  dimension "d15" = 19.05
  dimension "d16" = 19.05
  dimension "d17" = 19.05
  dimension "d18" = 57.15
  dimension "d19" = 19.05
  dimension "d20" = 19.05
  dimension "d21" = 19.05
  dimension "d22" = 57.15
  dimension "d23" = 19.05
  dimension "d24" = 23.81
  dimension "d25" = 19.05
  dimension "d26" = 23.81
  dimension "d27" = 19.05
  dimension "d28" = 19.05
  dimension "d29" = 19.05
  constraints: 212 end point, 44 parallel, 22 horizontal, 22 perpendicular, 18 midpoint, 695 other
  measures "d2" distance of L3730.end L3729.end
  measures "d3" distance of L3729.end L3728.end
  measures "d4" distance of L3740.end L3739.end
  measures "d5" distance of L3739.end L3738.end
  measures "d6" distance of L3745.end L3746.end
  measures "d7" distance of L3744.end L3745.end
  measures "d8" distance of L3754.end L3753.end
  measures "d9" distance of L3753.end L3752.end
  measures "d10" distance of L3763.end L3764.end
  measures "d11" distance of L3762.end L3763.end
  measures "d12" distance of L3771.end L3772.end
  measures "d13" distance of L3770.end L3771.end
  measures "d14" distance of L3777.end L3778.end
  measures "d15" distance of L3776.end L3777.end
  measures "d16" distance of L3782.end L3781.end
  measures "d17" distance of L3781.end L3780.end
  measures "d18" distance of L3787.end L3788.end
  measures "d19" distance of L3786.end L3787.end
  measures "d20" distance of L3792.end L3791.end
  measures "d21" distance of L3791.end L3790.end
  measures "d22" distance of L3797.end L3798.end
  measures "d23" distance of L3796.end L3797.end
  measures "d24" distance of L3802.end L3801.end
  measures "d25" distance of L3801.end L3800.end
  measures "d26" distance of L3812.end L3811.end
  measures "d27" distance of L3811.end L3810.end
  measures "d28" distance of L3822.end L3821.end
  measures "d29" distance of L3821.end L3820.end
sketch "Sketch4" plane through (0, 0, 1.5) normal (0, 0, 1) x (1, 0, 0)
  line L0 (0.3948, 100.5005) -> (19.4448, 100.5005) projected
  line L1 (19.4448, 100.5005) -> (19.4448, 119.5505) projected
  line L2 (38.4949, 100.5005) -> (38.4949, 119.5505) projected
  line L3 (57.5449, 100.5005) -> (38.4949, 100.5005) projected
  line L4 (114.6949, 100.5005) -> (57.5449, 100.5005) projected
  line L5 (19.4448, 95.7377) -> (248.0448, 95.7377) projected
  line L6 (19.4448, 95.7377) -> (0.3948, 95.7377) projected
  line L7 (114.6949, 119.5505) -> (114.6949, 100.5005) projected
  line L8 (119.458, 119.5505) -> (119.458, 100.5005) projected
  line L9 (119.458, 100.5005) -> (138.508, 100.5005) projected
  line L10 (195.658, 100.5005) -> (138.508, 100.5005) projected
  line L11 (195.658, 119.5505) -> (195.658, 100.5005) projected
  line L12 (200.4205, 119.5505) -> (200.4205, 100.5005) projected
  line L13 (200.4205, 100.5005) -> (219.4705, 100.5005) projected
  line L14 (276.6205, 100.5005) -> (219.4705, 100.5005) projected
  line L15 (276.6205, 119.5505) -> (276.6205, 100.5005) projected
  line L16 (286.1455, 95.7377) -> (248.0448, 95.7377) projected
  line L17 (305.1955, 95.7377) -> (286.1455, 95.7377) projected
  line L18 (248.0455, 19.5378) -> (238.5185, 19.5378) projected
  line L19 (248.0455, 19.5378) -> (248.0455, 0.4878) projected
  line L20 (238.5185, 0.4878) -> (238.5185, 19.5378) projected
  line L21 (0.0951, 117.85) -> (0.0951, 2.187) projected
  line L22 (303.496, 119.849) -> (2.096, 119.849) projected
  line L23 (305.496, 2.1869) -> (305.496, 117.85) projected
  line L24 (2.096, 0.1874) -> (303.496, 0.1874) projected
  line L25 (152.7955, 60.0182) -> (152.7955, 119.849)
  line L26 (152.7955, 60.0182) -> (152.7955, 0.1874)
  line L27 (152.7955, 60.0182) -> (305.496, 60.0185)
  line L28 (152.7955, 60.0182) -> (0.0951, 60.0182)
  line L29 (-12.2045, -14.4818) -> (317.7955, -14.4818)
  line L30 (317.7955, -14.4818) -> (317.7955, 134.5182)
  line L31 (317.7955, 134.5182) -> (-12.2045, 134.5182)
  line L32 (-12.2045, 134.5182) -> (-12.2045, -14.4818)
  line L33 (-12.2045, -14.4818) -> (317.7955, 134.5182) construction
  line L34 (317.7955, -14.4818) -> (-12.2045, 134.5182) construction
  line L35 (-5.5695, -7.8568) -> (311.1605, -7.8568)
  line L36 (311.1605, -7.8568) -> (311.1605, 127.8932)
  line L37 (311.1605, 127.8932) -> (-5.5695, 127.8932)
  line L38 (-5.5695, 127.8932) -> (-5.5695, -7.8568)
  line L39 (-5.5695, -7.8568) -> (311.1605, 127.8932) construction
  line L40 (311.1605, -7.8568) -> (-5.5695, 127.8932) construction
  line L41 (19.4448, 100.5005) -> (-12.2045, 100.5005)
  line L42 (-12.2045, 100.5005) -> (-12.2045, 134.5182)
  line L43 (-12.2045, 134.5182) -> (19.4448, 134.5182)
  line L44 (19.4448, 134.5182) -> (19.4448, 100.5005)
  line L45 (38.4949, 100.5005) -> (114.6949, 100.5005)
  line L46 (114.6949, 100.5005) -> (114.6949, 134.5182)
  line L47 (114.6949, 134.5182) -> (38.4949, 134.5182)
  line L48 (38.4949, 134.5182) -> (38.4949, 100.5005)
  line L49 (119.458, 100.5005) -> (195.658, 100.5005)
  line L50 (195.658, 100.5005) -> (195.658, 134.5182)
  line L51 (195.658, 134.5182) -> (119.458, 134.5182)
  line L52 (119.458, 134.5182) -> (119.458, 100.5005)
  line L53 (200.4205, 100.5005) -> (276.6205, 100.5005)
  line L54 (276.6205, 100.5005) -> (276.6205, 134.5182)
  line L55 (276.6205, 134.5182) -> (200.4205, 134.5182)
  line L56 (200.4205, 134.5182) -> (200.4205, 100.5005)
  line L57 (0.3948, 95.7377) -> (-12.2045, 95.7377)
  line L58 (305.1955, 95.7377) -> (317.7955, 95.7377)
  line L59 (238.5185, 19.5378) -> (248.0455, 19.5378)
  line L60 (248.0455, 19.5378) -> (248.0455, -14.4818)
  line L61 (248.0455, -14.4818) -> (238.5185, -14.4818)
  line L62 (238.5185, -14.4818) -> (238.5185, 19.5378)
  line L63 (0.0951, 100.5005) -> (305.496, 100.5005)
  line L64 (305.496, 100.5005) -> (305.496, 119.849)
  line L65 (305.496, 119.849) -> (0.0951, 119.849)
  line L66 (0.0951, 119.849) -> (0.0951, 100.5005)
  line L67 (0.0951, 119.849) -> (305.496, 119.849)
  line L68 (305.496, 119.849) -> (305.496, 0.1874)
  line L69 (305.496, 0.1874) -> (0.0951, 0.1874)
  line L70 (0.0951, 0.1874) -> (0.0951, 119.849)
  line L71 (-12.2045, 137.0582) -> (317.7923, 137.0582)
  line L72 (317.7923, 137.0582) -> (317.7923, -11.9382)
  line L73 (317.7923, -11.9382) -> (-12.2045, -11.9382)
  line L74 (-12.2045, -11.9382) -> (-12.2045, 137.0582)
  point P0 (0, 0)
  point P1 (305.496, 60.0185)
  point P2 (38.4949, 119.849)
  point P3 (114.6949, 119.849)
  point P4 (0.0951, 95.7377)
  point P5 (305.496, 95.7377)
  point P6 (248.0455, 0.1874)
  point P7 (238.5185, 0.1874)
  point P8 (19.4448, 119.849)
  point P9 (2.096, 119.849)
  point P10 (200.4205, 119.849)
  point P11 (276.6205, 119.849)
  point P12 (119.458, 119.849)
  point P13 (195.658, 119.849)
  point P14 (-12.2045, -11.9382)
  point P15 (317.7923, 95.7377)
  point P16 (317.7923, 134.5182)
  dimension "d34" = 330
  dimension "d35" = 149
  dimension "d36" = 316.73
  dimension "d37" = 135.75
  dimension "d40" = 329.9968
  dimension "d41" = 148.9964
  dimension "d42" = 0
  dimension "d43" = 2.54
  constraints: 100 end point, 20 parallel, 16 point on line, 14 perpendicular, 10 horizontal, 6 midpoint, 2 equal length
  measures "d34" distance of L31.end L30.end
  measures "d35" distance of L30.end L29.end
  measures "d36" distance of L37.end L36.end
  measures "d37" distance of L37.end L35.start
  measures "d40" distance of L72.end L73.end
  measures "d41" distance of L71.end L72.end
  measures "d42" distance between parallel lines of L74 L32
  measures "d43" distance between parallel lines of L71 L31
extrude "Extrusion3" add sketch "Sketch4" along normal blind 10 contours L0 L63 L3 L4 L9 L10 L25 L5 L6 L57 L21 L41 | L1 L44 L22 L48 L2 L63 | L41 L38 L37 L44 L22 L65 L66 L21 | L21 L57 L38 L41 | L21 L70 L69 L24 L62 L35 L38 L57 | L41 L32 L31 L44 L37 L38 | L38 L57 L32 L41 | L44 L37 L48 L22 | L38 L35 L62 L73 L32 L57 | L48 L37 L46 L22 | L44 L31 L48 L37 | L7 L46 L22 L52 L8 L63 | L74 L71 L72 L31 | L46 L37 L52 L22 | L48 L31 L46 L37 | L25 L10 L63 L13 L14 L23 L58 L17 L16 L5 | L23 L58 L36 L35 L60 L24 L69 L68 | L62 L24 L60 L35 | L35 L60 L73 L62 | L52 L37 L50 L22 | L46 L31 L52 L37 | L62 L20 L18 L19 L60 L24 | L23 L64 L65 L22 L54 L37 L36 L58 | L35 L36 L58 L72 L73 L60 | L52 L31 L50 L37 | L11 L50 L22 L56 L12 L63 | L63 L15 L54 L22 L65 L64 L23 | L36 L37 L54 L31 L72 L58 | L31 L30 L58 L72 | L50 L37 L56 L22 | L50 L31 L56 L37 | L54 L37 L56 L31 | L56 L37 L54 L22
sketch "Sketch5" plane through (0, 0, 1.5) normal (0, 0, -1) x (-1, 0, 0)
  line L0 (-317.7923, 134.5182) -> (-317.7923, 137.0582) projected
  line L1 (12.2045, -11.9382) -> (-317.7923, -11.9382)
  line L2 (-317.7923, -11.9382) -> (-317.7923, 137.0582)
  line L3 (-317.7923, 137.0582) -> (12.2045, 137.0582)
  line L4 (12.2045, 137.0582) -> (12.2045, -11.9382)
  line L5 (-311.1589, 130.435) -> (5.5711, 130.435)
  line L6 (5.5711, 130.435) -> (5.5711, -5.315)
  line L7 (5.5711, -5.315) -> (-311.1589, -5.315)
  line L8 (-311.1589, -5.315) -> (-311.1589, 130.435)
  line L9 (-311.1589, 130.435) -> (5.5711, -5.315) construction
  line L10 (5.5711, 130.435) -> (-311.1589, -5.315) construction
  point P0 (0, 0)
  point P1 (-152.7939, 62.56)
  dimension "d44" = 316.73
  dimension "d45" = 135.75
  constraints: 20 end point, 4 parallel, 2 horizontal, 2 midpoint, 2 perpendicular
  measures "d44" distance of L6.end L7.end
  measures "d45" distance of L7.end L5.start
extrude "Extrusion4" cut sketch "Sketch5" against normal blind 3 contours L5 L6 L7 L8
fillet "Fillet1" radius 2 4 edges at (-12.2045, 137.0582, 6.5) (317.7923, 137.0582, 6.5) (317.7923, -11.9382, 6.5) (-12.2045, -11.9382, 6.5)
body "Solid2"
